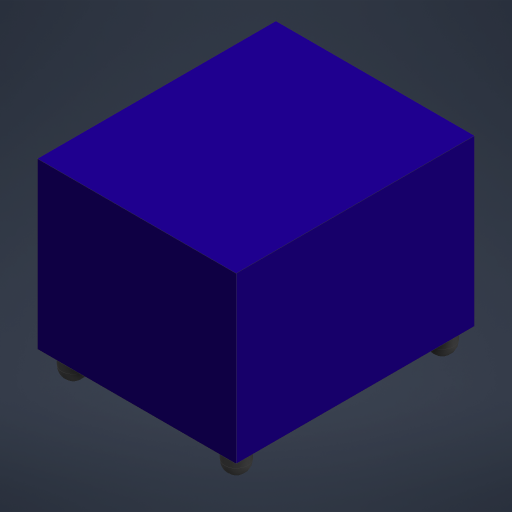
# Autodesk Inventor part: PXie-1083
Saved by Autodesk Inventor 2024.3 (Build 283343000, 343)
## iProperties
Created: 2024-06-12
Part Number: PXie-1083
Material: Generic
Document SubType Name: Modeling
Designer: braed
Density: 1 g/cm^3
Appearance: Default
Author: braed
Autodesk Inventor part; units mm, degrees
ref_plane "YZ Plane" through (0, 0, 0) normal (1, 0, 0) x (0, 1, 0)
ref_plane "XZ Plane" through (0, 0, 0) normal (0, 1, 0) x (-1, 0, 0)
ref_plane "XY Plane" through (0, 0, 0) normal (0, 0, 1) x (1, 0, 0)
sketch "Sketch1" plane through (0, 0, 0) normal (0, 0, 1) x (1, 0, 0)
  line L0 (0, 0) -> (214.3125, 0)
  line L1 (214.3125, 0) -> (214.3125, 177.8)
  line L2 (214.3125, 177.8) -> (0, 177.8)
  line L3 (0, 177.8) -> (0, 0)
  dimension "d0" = 214.3125
  dimension "d1" = 177.8
  constraints: 8 end point, 2 parallel, 1 horizontal, 1 perpendicular
  measures "d0" distance of L2.end L1.end
  measures "d1" distance of L1.end L0.end
extrude "Extrusion1" add sketch "Sketch1" along normal blind 257.175
sketch "Sketch2" plane through (0, 0, 0) normal (0, -1, 0) x (1, 0, 0)
  line L0 (214.3125, 0) -> (214.3125, 257.175) projected
  line L1 (214.3125, 128.5875) -> (107.1562, 128.5875) construction
  line L2 (107.1562, 128.5875) -> (107.1562, 0) construction
  line L3 (214.3125, 257.175) -> (0, 257.175) construction
  line L4 (214.3125, 0) -> (214.3125, 257.175) construction
  line L5 (214.3125, 257.175) -> (214.3125, 239.649) construction
  line L6 (214.3125, 239.649) -> (196.9389, 239.649) construction
  circle A0 centre (196.9389, 239.649) radius 12.7
  circle A1 centre (196.9389, 17.526) radius 12.7
  line L7 (196.9389, 239.649) -> (11.3133, 239.649) construction
  circle A2 centre (21.2344, 239.649) radius 12.7
  line L8 (0, 0) -> (0, 257.175) construction
  circle A3 centre (21.2344, 17.526) radius 12.7
  dimension "d4" = 107.1562
  dimension "d6" = 17.526
  dimension "d7" = 17.3736
  dimension "d8" = 25.4
  dimension "d9" = 25.4
  dimension "d10" = 21.2344
  constraints: 10 end point, 4 centre point, 3 horizontal, 2 point on line, 2 symmetric about line, 1 coincident, 1 midpoint, 1 vertical, 2 other
  measures "d4" distance of L1.start L1.end
  measures "d6" distance of L0.end L5.end
  measures "d7" distance of L5.end L6.end
  measures "d8" diameter of A0
  measures "d9" diameter of A2
  measures "d10" distance from line of L8 A2.centre
extrude "Extrusion2" add sketch "Sketch2" along normal blind 25.4
fillet "Fillet1" radius 12.7 4 edges at (184.2389, -25.4, 239.649) (8.5344, -25.4, 239.649) (8.5344, -25.4, 17.526) (184.2389, -25.4, 17.526)
sketch "Sketch3" plane through (0, 0, 0) normal (-1, 0, 0) x (0, 0, 1)
  line L0 (257.175, 0) -> (257.175, 177.8) projected
  line L1 (257.175, 177.8) -> (257.175, 165.1)
  line L2 (257.175, 165.1) -> (244.475, 165.1)
  line L3 (0, 0) -> (101.6, 0)
  line L4 (101.6, 0) -> (101.6, 12.7)
  line L5 (244.475, 165.1) -> (101.6, 165.1)
  line L6 (101.6, 165.1) -> (101.6, 12.7)
  line L7 (101.6, 12.7) -> (244.475, 12.7)
  line L8 (244.475, 12.7) -> (244.475, 165.1)
  dimension "d14" = 12.7
  dimension "d15" = 12.7
  dimension "d16" = 101.6
  dimension "d17" = 12.7
  constraints: 16 end point, 3 perpendicular, 2 horizontal, 2 parallel, 1 point on line
  measures "d14" distance of L0.end L1.end
  measures "d15" distance of L1.end L2.end
  measures "d16" distance of L3.start L3.end
  measures "d17" distance of L3.end L4.end
extrude "Extrusion3" cut sketch "Sketch3" against normal blind 10.16
body "Solid1"
